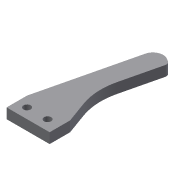
# Autodesk Inventor part: gripper
Saved by Autodesk Inventor 2018 (Build 220112000, 112)
## iProperties
Created: 2016-10-14
Part Number: gripper
Material: Generic
Document SubType Name: Modeling
Designer: Bardo91
Density: 1 g/cm^3
Appearance: Default
Author: Bardo91
Autodesk Inventor part; units mm, degrees
ref_plane "YZ Plane" through (0, 0, 0) normal (1, 0, 0) x (0, 1, 0)
ref_plane "XZ Plane" through (0, 0, 0) normal (0, 1, 0) x (-1, 0, 0)
ref_plane "XY Plane" through (0, 0, 0) normal (0, 0, 1) x (1, 0, 0)
sketch "Sketch1" plane through (0, 0, 0) normal (0, 0, 1) x (1, 0, 0)
  line L0 (0, 0) -> (5, 0)
  line L1 (5, 0) -> (-5, 0)
  circle A0 centre (-5, 0) radius 1.75
  circle A1 centre (5, 0) radius 1.75
  line L2 (0, 0) -> (0, -5)
  line L3 (0, -5) -> (11, -5)
  line L4 (11, -5) -> (11, 5)
  line L5 (0, -5) -> (-10, -5)
  line L6 (-10, -5) -> (-10, 5)
  line L7 (11, 5) -> (7.2436, 15.3207)
  line L8 (11, 5) -> (21.9831, 5) construction
  line L9 (6.2581, 32.5632) -> (10.8155, 51.6081)
  line L10 (9.9731, 53.7422) -> (8.756, 54.5465)
  line L11 (1.1367, 51.5387) -> (-10, 5)
  arc A2 (6.2581, 32.5632) -> (7.2436, 15.3207) centre (35.4343, 25.5813) ccw
  arc A3 (10.8155, 51.6081) -> (9.9731, 53.7422) centre (8.8705, 52.0736) ccw
  arc A4 (8.756, 54.5465) -> (1.1367, 51.5387) centre (5.9994, 50.375) ccw
  point P0 (4.1596, 23.7939)
  point P1 (11.1415, 52.9701)
  point P2 (2.7985, 58.4833)
  dimension "d0" = 5
  dimension "d1" = 10
  dimension "d2" = 3.5
  dimension "d3" = 3.5
  dimension "d4" = 5
  dimension "d5" = 11
  dimension "d6" = 10
  dimension "d7" = 10
  dimension "d8" = 10
  dimension "d9" = 20
  dimension "d10" = 110
  dimension "d11" = 30
  dimension "d12" = 10
  dimension "d13" = 110
  dimension "d14" = 30
  dimension "d15" = 2
  dimension "d16" = 5
  constraints: 24 end point, 7 point on line, 6 point on circle, 6 tangent, 5 centre point, 3 horizontal, 3 perpendicular, 2 coincident, 1 equal length, 1 parallel, 1 vertical
  measures "d0" distance of L0.start L0.end
  measures "d1" distance of L0.end L1.end
  measures "d2" diameter of A0
  measures "d3" diameter of A1
  measures "d4" distance of L0.start L2.end
  measures "d5" distance of L2.end L3.end
  measures "d6" distance of L3.end L4.end
  measures "d7" distance of L2.end L5.end
  measures "d8" distance of L5.end L6.end
  measures "d9" distance of L4.end point (4.16, 23.794)
  measures "d10" angle of L8 L7
  measures "d11" distance of point (4.16, 23.794) point (11.141, 52.97)
  measures "d12" distance of point (11.141, 52.97) point (2.799, 58.483)
  measures "d13" angle of L10 L9
  measures "d14" radius of A2
  measures "d15" radius of A3
  measures "d16" radius of A4
extrude "Extrusion1" add sketch "Sketch1" along normal blind 5
body "Solid1"
